Autodesk Inventor part; units mm, degrees
(part 4 of 4)
sketch "Sketch20" plane through (0, 0, 0) normal (0, 0, -1) x (-1, 0, 0)
  line L0 (-13.5496, 2.1542) -> (-13.5496, 4.2325)
  line L1 (-14.7777, 4.2325) -> (-14.7777, 2.1542)
  line L2 (-14.7777, 4.2325) -> (-13.5496, 4.2325)
  line L3 (-13.5496, 4.2325) -> (-13.0496, 4.2325)
  line L4 (-13.0496, 4.2325) -> (-13.0496, 3.7325)
  line L5 (-13.0496, 3.7325) -> (-13.5496, 3.7325)
  line L6 (-13.5496, 2.1542) -> (-13.0496, 2.1542)
  line L7 (-13.0496, 2.1542) -> (-13.0496, 2.6542)
  line L8 (-13.0496, 2.6542) -> (-13.5496, 2.6542)
  line L9 (-14.7777, 2.1542) -> (-14.7777, 4.2325)
  line L10 (-15.2777, 3.1933) -> (-15.2777, 3.4433)
  line L11 (-15.2777, 3.4433) -> (-14.7777, 3.4433)
  line L12 (-15.2777, 3.1933) -> (-15.2777, 2.9433)
  line L13 (-15.2777, 2.9433) -> (-14.7777, 2.9433)
  point P0 (0, 0)
  dimension "d129" = 0.5
  dimension "d130" = 0.5
  dimension "d131" = 0.5
  dimension "d132" = 0.5
  dimension "d134" = 0.25
  dimension "d135" = 0.25
  constraints: 20 end point, 6 point on line, 5 perpendicular, 2 vertical, 1 horizontal
  measures "d129" distance of L0.end L3.end
  measures "d130" distance of L3.end L4.end
  measures "d131" distance of L0.start L6.end
  measures "d132" distance of L6.end L7.end
  measures "d134" distance of L10.start L10.end
  measures "d135" distance of L10.start L12.end
extrude "Extrusion20" add sketch "Sketch20" along normal blind 0.5 separate body
chamfer "Chamfer7" distance 0.3 angle 45 3 edges at (13.0496, 3.9825, -0.5) (13.0496, 2.4042, -0.5) (15.2777, 3.1933, -0.5)
body "Solid1"
body "Solid2"
body "Solid3"
body "Solid4"
body "Solid5"
body "Solid6"
body "Solid7"
body "Solid8"
body "Solid9"
body "Solid10"
body "Solid11"
body "Solid12"
body "Solid13"
body "Solid14"
body "Solid15"
body "Solid16"
body "Solid17"
